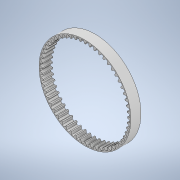
# Autodesk Inventor part: Zahnriemen
Saved by Autodesk Inventor 2021 (Build 250183000, 183)
## iProperties
Created: 2021-08-21
Part Number: Zahnriemen
Material: Generisch
Document SubType Name: Modeling
Designer: stroh
Density: 1 g/cm^3
Appearance: Vorgabe
Author: stroh
Autodesk Inventor part; units mm, degrees
ref_plane "YZ Plane" through (0, 0, 0) normal (1, 0, 0) x (0, 1, 0)
ref_plane "XZ Plane" through (0, 0, 0) normal (0, 1, 0) x (-1, 0, 0)
ref_plane "XY Plane" through (0, 0, 0) normal (0, 0, 1) x (1, 0, 0)
sketch "Skizze2" plane through (0, 0, 0) normal (0, 0, 1) x (1, 0, 0)
  circle A0 centre (0, 0) radius 44.5634
  line L0 (1.5, 44.5381) -> (0.5, 42.0381)
  line L1 (0.5, 42.0381) -> (-0.5, 42.0381)
  line L2 (-0.5, 42.0381) -> (-1.5, 44.5381)
  arc A1 (1.5, 44.5381) -> (-1.5, 44.5381) centre (0, 0) ccw
  circle A2 centre (0, 0) radius 45.5
  arc A3 (-3.4961, 44.426) -> (-6.4773, 44.0901) centre (0, 0) ccw
  line L3 (-5.2036, 41.7178) -> (-6.4773, 44.0901)
  line L4 (-4.2099, 41.8298) -> (-5.2036, 41.7178)
  line L5 (-3.4961, 44.426) -> (-4.2099, 41.8298)
  arc A4 (-8.4483, 43.7553) -> (-11.3731, 43.0877) centre (0, 0) ccw
  line L6 (-9.8418, 40.8729) -> (-11.3731, 43.0877)
  line L7 (-8.8669, 41.0954) -> (-9.8418, 40.8729)
  line L8 (-8.4483, 43.7553) -> (-8.8669, 41.0954)
  arc A5 (-13.2942, 42.5342) -> (-16.1258, 41.5434) centre (0, 0) ccw
  line L9 (-14.3563, 39.514) -> (-16.1258, 41.5434)
  line L10 (-13.4124, 39.8442) -> (-14.3563, 39.514)
  line L11 (-13.2942, 42.5342) -> (-13.4124, 39.8442)
  arc A6 (-17.9729, 40.7783) -> (-20.6758, 39.4766) centre (0, 0) ccw
  line L12 (-18.6901, 37.6581) -> (-20.6758, 39.4766)
  line L13 (-17.7892, 38.092) -> (-18.6901, 37.6581)
  line L14 (-17.9729, 40.7783) -> (-17.7892, 38.092)
  arc A7 (-22.4256, 38.5096) -> (-24.9658, 36.9135) centre (0, 0) ccw
  line L15 (-22.789, 35.3287) -> (-24.9658, 36.9135)
  line L16 (-21.9423, 35.8607) -> (-22.789, 35.3287)
  line L17 (-22.4256, 38.5096) -> (-21.9423, 35.8607)
  arc A8 (-26.5963, 35.7565) -> (-28.9418, 33.8861) centre (0, 0) ccw
  line L18 (-26.6013, 32.555) -> (-28.9418, 33.8861)
  line L19 (-25.8194, 33.1785) -> (-26.6013, 32.555)
  line L20 (-26.5963, 35.7565) -> (-25.8194, 33.1785)
  arc A9 (-30.4326, 32.5539) -> (-32.5539, 30.4326) centre (0, 0) ccw
  line L21 (-30.079, 29.3719) -> (-32.5539, 30.4326)
  line L22 (-29.3719, 30.079) -> (-30.079, 29.3719)
  line L23 (-30.4326, 32.5539) -> (-29.3719, 30.079)
  arc A10 (-33.8861, 28.9418) -> (-35.7565, 26.5963) centre (0, 0) ccw
  line L24 (-33.1785, 25.8194) -> (-35.7565, 26.5963)
  line L25 (-32.555, 26.6013) -> (-33.1785, 25.8194)
  line L26 (-33.8861, 28.9418) -> (-32.555, 26.6013)
  arc A11 (-36.9135, 24.9658) -> (-38.5096, 22.4256) centre (0, 0) ccw
  line L27 (-35.8607, 21.9423) -> (-38.5096, 22.4256)
  line L28 (-35.3287, 22.789) -> (-35.8607, 21.9423)
  line L29 (-36.9135, 24.9658) -> (-35.3287, 22.789)
  arc A12 (-39.4766, 20.6758) -> (-40.7783, 17.9729) centre (0, 0) ccw
  line L30 (-38.092, 17.7892) -> (-40.7783, 17.9729)
  line L31 (-37.6581, 18.6901) -> (-38.092, 17.7892)
  line L32 (-39.4766, 20.6758) -> (-37.6581, 18.6901)
  arc A13 (-41.5434, 16.1258) -> (-42.5342, 13.2942) centre (0, 0) ccw
  line L33 (-39.8442, 13.4124) -> (-42.5342, 13.2942)
  line L34 (-39.514, 14.3563) -> (-39.8442, 13.4124)
  line L35 (-41.5434, 16.1258) -> (-39.514, 14.3563)
  arc A14 (-43.0877, 11.3731) -> (-43.7553, 8.4483) centre (0, 0) ccw
  line L36 (-41.0954, 8.8669) -> (-43.7553, 8.4483)
  line L37 (-40.8729, 9.8418) -> (-41.0954, 8.8669)
  line L38 (-43.0877, 11.3731) -> (-40.8729, 9.8418)
  arc A15 (-44.0901, 6.4773) -> (-44.426, 3.4961) centre (0, 0) ccw
  line L39 (-41.8298, 4.2099) -> (-44.426, 3.4961)
  line L40 (-41.7178, 5.2036) -> (-41.8298, 4.2099)
  line L41 (-44.0901, 6.4773) -> (-41.7178, 5.2036)
  arc A16 (-44.5381, 1.5) -> (-44.5381, -1.5) centre (0, 0) ccw
  line L42 (-42.0381, -0.5) -> (-44.5381, -1.5)
  line L43 (-42.0381, 0.5) -> (-42.0381, -0.5)
  line L44 (-44.5381, 1.5) -> (-42.0381, 0.5)
  arc A17 (-44.426, -3.4961) -> (-44.0901, -6.4773) centre (0, 0) ccw
  line L45 (-41.7178, -5.2036) -> (-44.0901, -6.4773)
  line L46 (-41.8298, -4.2099) -> (-41.7178, -5.2036)
  line L47 (-44.426, -3.4961) -> (-41.8298, -4.2099)
  arc A18 (-43.7553, -8.4483) -> (-43.0877, -11.3731) centre (0, 0) ccw
  line L48 (-40.8729, -9.8418) -> (-43.0877, -11.3731)
  line L49 (-41.0954, -8.8669) -> (-40.8729, -9.8418)
  line L50 (-43.7553, -8.4483) -> (-41.0954, -8.8669)
  arc A19 (-42.5342, -13.2942) -> (-41.5434, -16.1258) centre (0, 0) ccw
  line L51 (-39.514, -14.3563) -> (-41.5434, -16.1258)
  line L52 (-39.8442, -13.4124) -> (-39.514, -14.3563)
  line L53 (-42.5342, -13.2942) -> (-39.8442, -13.4124)
  arc A20 (-40.7783, -17.9729) -> (-39.4766, -20.6758) centre (0, 0) ccw
  line L54 (-37.6581, -18.6901) -> (-39.4766, -20.6758)
  line L55 (-38.092, -17.7892) -> (-37.6581, -18.6901)
  line L56 (-40.7783, -17.9729) -> (-38.092, -17.7892)
  arc A21 (-38.5096, -22.4256) -> (-36.9135, -24.9658) centre (0, 0) ccw
  line L57 (-35.3287, -22.789) -> (-36.9135, -24.9658)
  line L58 (-35.8607, -21.9423) -> (-35.3287, -22.789)
  line L59 (-38.5096, -22.4256) -> (-35.8607, -21.9423)
  arc A22 (-35.7565, -26.5963) -> (-33.8861, -28.9418) centre (0, 0) ccw
  line L60 (-32.555, -26.6013) -> (-33.8861, -28.9418)
  line L61 (-33.1785, -25.8194) -> (-32.555, -26.6013)
  line L62 (-35.7565, -26.5963) -> (-33.1785, -25.8194)
  arc A23 (-32.5539, -30.4326) -> (-30.4326, -32.5539) centre (0, 0) ccw
  line L63 (-29.3719, -30.079) -> (-30.4326, -32.5539)
  line L64 (-30.079, -29.3719) -> (-29.3719, -30.079)
  line L65 (-32.5539, -30.4326) -> (-30.079, -29.3719)
  arc A24 (-28.9418, -33.8861) -> (-26.5963, -35.7565) centre (0, 0) ccw
  line L66 (-25.8194, -33.1785) -> (-26.5963, -35.7565)
  line L67 (-26.6013, -32.555) -> (-25.8194, -33.1785)
  line L68 (-28.9418, -33.8861) -> (-26.6013, -32.555)
  arc A25 (-24.9658, -36.9135) -> (-22.4256, -38.5096) centre (0, 0) ccw
  line L69 (-21.9423, -35.8607) -> (-22.4256, -38.5096)
  line L70 (-22.789, -35.3287) -> (-21.9423, -35.8607)
  line L71 (-24.9658, -36.9135) -> (-22.789, -35.3287)
  arc A26 (-20.6758, -39.4766) -> (-17.9729, -40.7783) centre (0, 0) ccw
  line L72 (-17.7892, -38.092) -> (-17.9729, -40.7783)
  line L73 (-18.6901, -37.6581) -> (-17.7892, -38.092)
  line L74 (-20.6758, -39.4766) -> (-18.6901, -37.6581)
  arc A27 (-16.1258, -41.5434) -> (-13.2942, -42.5342) centre (0, 0) ccw
  line L75 (-13.4124, -39.8442) -> (-13.2942, -42.5342)
  line L76 (-14.3563, -39.514) -> (-13.4124, -39.8442)
  line L77 (-16.1258, -41.5434) -> (-14.3563, -39.514)
  arc A28 (-11.3731, -43.0877) -> (-8.4483, -43.7553) centre (0, 0) ccw
  line L78 (-8.8669, -41.0954) -> (-8.4483, -43.7553)
  line L79 (-9.8418, -40.8729) -> (-8.8669, -41.0954)
  line L80 (-11.3731, -43.0877) -> (-9.8418, -40.8729)
  arc A29 (-6.4773, -44.0901) -> (-3.4961, -44.426) centre (0, 0) ccw
  line L81 (-4.2099, -41.8298) -> (-3.4961, -44.426)
  line L82 (-5.2036, -41.7178) -> (-4.2099, -41.8298)
  line L83 (-6.4773, -44.0901) -> (-5.2036, -41.7178)
  arc A30 (-1.5, -44.5381) -> (1.5, -44.5381) centre (0, 0) ccw
  line L84 (0.5, -42.0381) -> (1.5, -44.5381)
  line L85 (-0.5, -42.0381) -> (0.5, -42.0381)
  line L86 (-1.5, -44.5381) -> (-0.5, -42.0381)
  arc A31 (3.4961, -44.426) -> (6.4773, -44.0901) centre (0, 0) ccw
  line L87 (5.2036, -41.7178) -> (6.4773, -44.0901)
  line L88 (4.2099, -41.8298) -> (5.2036, -41.7178)
  line L89 (3.4961, -44.426) -> (4.2099, -41.8298)
  arc A32 (8.4483, -43.7553) -> (11.3731, -43.0877) centre (0, 0) ccw
  line L90 (9.8418, -40.8729) -> (11.3731, -43.0877)
  line L91 (8.8669, -41.0954) -> (9.8418, -40.8729)
  line L92 (8.4483, -43.7553) -> (8.8669, -41.0954)
  arc A33 (13.2942, -42.5342) -> (16.1258, -41.5434) centre (0, 0) ccw
  line L93 (14.3563, -39.514) -> (16.1258, -41.5434)
  line L94 (13.4124, -39.8442) -> (14.3563, -39.514)
  line L95 (13.2942, -42.5342) -> (13.4124, -39.8442)
  arc A34 (17.9729, -40.7783) -> (20.6758, -39.4766) centre (0, 0) ccw
  line L96 (18.6901, -37.6581) -> (20.6758, -39.4766)
  line L97 (17.7892, -38.092) -> (18.6901, -37.6581)
  line L98 (17.9729, -40.7783) -> (17.7892, -38.092)
  arc A35 (22.4256, -38.5096) -> (24.9658, -36.9135) centre (0, 0) ccw
  line L99 (22.789, -35.3287) -> (24.9658, -36.9135)
  line L100 (21.9423, -35.8607) -> (22.789, -35.3287)
  line L101 (22.4256, -38.5096) -> (21.9423, -35.8607)
  arc A36 (26.5963, -35.7565) -> (28.9418, -33.8861) centre (0, 0) ccw
  line L102 (26.6013, -32.555) -> (28.9418, -33.8861)
  line L103 (25.8194, -33.1785) -> (26.6013, -32.555)
  line L104 (26.5963, -35.7565) -> (25.8194, -33.1785)
  arc A37 (30.4326, -32.5539) -> (32.5539, -30.4326) centre (0, 0) ccw
  line L105 (30.079, -29.3719) -> (32.5539, -30.4326)
  line L106 (29.3719, -30.079) -> (30.079, -29.3719)
  line L107 (30.4326, -32.5539) -> (29.3719, -30.079)
  arc A38 (33.8861, -28.9418) -> (35.7565, -26.5963) centre (0, 0) ccw
  line L108 (33.1785, -25.8194) -> (35.7565, -26.5963)
  line L109 (32.555, -26.6013) -> (33.1785, -25.8194)
  line L110 (33.8861, -28.9418) -> (32.555, -26.6013)
  arc A39 (36.9135, -24.9658) -> (38.5096, -22.4256) centre (0, 0) ccw
  line L111 (35.8607, -21.9423) -> (38.5096, -22.4256)
  line L112 (35.3287, -22.789) -> (35.8607, -21.9423)
  line L113 (36.9135, -24.9658) -> (35.3287, -22.789)
  arc A40 (39.4766, -20.6758) -> (40.7783, -17.9729) centre (0, 0) ccw
  line L114 (38.092, -17.7892) -> (40.7783, -17.9729)
  line L115 (37.6581, -18.6901) -> (38.092, -17.7892)
  line L116 (39.4766, -20.6758) -> (37.6581, -18.6901)
  arc A41 (41.5434, -16.1258) -> (42.5342, -13.2942) centre (0, 0) ccw
  line L117 (39.8442, -13.4124) -> (42.5342, -13.2942)
  line L118 (39.514, -14.3563) -> (39.8442, -13.4124)
  line L119 (41.5434, -16.1258) -> (39.514, -14.3563)
  arc A42 (43.0877, -11.3731) -> (43.7553, -8.4483) centre (0, 0) ccw
  line L120 (41.0954, -8.8669) -> (43.7553, -8.4483)
  line L121 (40.8729, -9.8418) -> (41.0954, -8.8669)
  line L122 (43.0877, -11.3731) -> (40.8729, -9.8418)
  arc A43 (44.0901, -6.4773) -> (44.426, -3.4961) centre (0, 0) ccw
  line L123 (41.8298, -4.2099) -> (44.426, -3.4961)
  line L124 (41.7178, -5.2036) -> (41.8298, -4.2099)
  line L125 (44.0901, -6.4773) -> (41.7178, -5.2036)
  arc A44 (44.5381, -1.5) -> (44.5381, 1.5) centre (0, 0) ccw
  line L126 (42.0381, 0.5) -> (44.5381, 1.5)
  line L127 (42.0381, -0.5) -> (42.0381, 0.5)
  line L128 (44.5381, -1.5) -> (42.0381, -0.5)
  arc A45 (44.426, 3.4961) -> (44.0901, 6.4773) centre (0, 0) ccw
  line L129 (41.7178, 5.2036) -> (44.0901, 6.4773)
  line L130 (41.8298, 4.2099) -> (41.7178, 5.2036)
  line L131 (44.426, 3.4961) -> (41.8298, 4.2099)
  arc A46 (43.7553, 8.4483) -> (43.0877, 11.3731) centre (0, 0) ccw
  line L132 (40.8729, 9.8418) -> (43.0877, 11.3731)
  line L133 (41.0954, 8.8669) -> (40.8729, 9.8418)
  line L134 (43.7553, 8.4483) -> (41.0954, 8.8669)
  arc A47 (42.5342, 13.2942) -> (41.5434, 16.1258) centre (0, 0) ccw
  line L135 (39.514, 14.3563) -> (41.5434, 16.1258)
  line L136 (39.8442, 13.4124) -> (39.514, 14.3563)
  line L137 (42.5342, 13.2942) -> (39.8442, 13.4124)
  arc A48 (40.7783, 17.9729) -> (39.4766, 20.6758) centre (0, 0) ccw
  line L138 (37.6581, 18.6901) -> (39.4766, 20.6758)
  line L139 (38.092, 17.7892) -> (37.6581, 18.6901)
  line L140 (40.7783, 17.9729) -> (38.092, 17.7892)
  arc A49 (38.5096, 22.4256) -> (36.9135, 24.9658) centre (0, 0) ccw
  line L141 (35.3287, 22.789) -> (36.9135, 24.9658)
  line L142 (35.8607, 21.9423) -> (35.3287, 22.789)
  line L143 (38.5096, 22.4256) -> (35.8607, 21.9423)
  arc A50 (35.7565, 26.5963) -> (33.8861, 28.9418) centre (0, 0) ccw
  line L144 (32.555, 26.6013) -> (33.8861, 28.9418)
  line L145 (33.1785, 25.8194) -> (32.555, 26.6013)
  line L146 (35.7565, 26.5963) -> (33.1785, 25.8194)
  arc A51 (32.5539, 30.4326) -> (30.4326, 32.5539) centre (0, 0) ccw
  line L147 (29.3719, 30.079) -> (30.4326, 32.5539)
  line L148 (30.079, 29.3719) -> (29.3719, 30.079)
  line L149 (32.5539, 30.4326) -> (30.079, 29.3719)
  arc A52 (28.9418, 33.8861) -> (26.5963, 35.7565) centre (0, 0) ccw
  line L150 (25.8194, 33.1785) -> (26.5963, 35.7565)
  line L151 (26.6013, 32.555) -> (25.8194, 33.1785)
  line L152 (28.9418, 33.8861) -> (26.6013, 32.555)
  arc A53 (24.9658, 36.9135) -> (22.4256, 38.5096) centre (0, 0) ccw
  line L153 (21.9423, 35.8607) -> (22.4256, 38.5096)
  line L154 (22.789, 35.3287) -> (21.9423, 35.8607)
  line L155 (24.9658, 36.9135) -> (22.789, 35.3287)
  arc A54 (20.6758, 39.4766) -> (17.9729, 40.7783) centre (0, 0) ccw
  line L156 (17.7892, 38.092) -> (17.9729, 40.7783)
  line L157 (18.6901, 37.6581) -> (17.7892, 38.092)
  line L158 (20.6758, 39.4766) -> (18.6901, 37.6581)
  arc A55 (16.1258, 41.5434) -> (13.2942, 42.5342) centre (0, 0) ccw
  line L159 (13.4124, 39.8442) -> (13.2942, 42.5342)
  line L160 (14.3563, 39.514) -> (13.4124, 39.8442)
  line L161 (16.1258, 41.5434) -> (14.3563, 39.514)
  arc A56 (11.3731, 43.0877) -> (8.4483, 43.7553) centre (0, 0) ccw
  line L162 (8.8669, 41.0954) -> (8.4483, 43.7553)
  line L163 (9.8418, 40.8729) -> (8.8669, 41.0954)
  line L164 (11.3731, 43.0877) -> (9.8418, 40.8729)
  arc A57 (6.4773, 44.0901) -> (3.4961, 44.426) centre (0, 0) ccw
  line L165 (4.2099, 41.8298) -> (3.4961, 44.426)
  line L166 (5.2036, 41.7178) -> (4.2099, 41.8298)
  line L167 (6.4773, 44.0901) -> (5.2036, 41.7178)
  point P0 (44.5381, 1.5)
  point P1 (44.5381, -1.5)
  point P2 (44.426, -3.4961)
  point P3 (44.0901, -6.4773)
  point P4 (43.7553, -8.4483)
  point P5 (43.0877, -11.3731)
  point P6 (42.5342, -13.2942)
  point P7 (41.5434, -16.1258)
  point P8 (40.7783, -17.9729)
  point P9 (39.4766, -20.6758)
  point P10 (38.5096, -22.4256)
  point P11 (36.9135, -24.9658)
  point P12 (35.7565, -26.5963)
  point P13 (33.8861, -28.9418)
  point P14 (32.5539, -30.4326)
  point P15 (30.4326, -32.5539)
  point P16 (28.9418, -33.8861)
  point P17 (26.5963, -35.7565)
  point P18 (24.9658, -36.9135)
  point P19 (22.4256, -38.5096)
  point P20 (20.6758, -39.4766)
  point P21 (17.9729, -40.7783)
  point P22 (16.1258, -41.5434)
  point P23 (13.2942, -42.5342)
  point P24 (11.3731, -43.0877)
  point P25 (8.4483, -43.7553)
  point P26 (6.4773, -44.0901)
  point P27 (3.4961, -44.426)
  point P28 (1.5, -44.5381)
  point P29 (-1.5, -44.5381)
  point P30 (-3.4961, -44.426)
  point P31 (-6.4773, -44.0901)
  point P32 (-8.4483, -43.7553)
  point P33 (-11.3731, -43.0877)
  point P34 (-13.2942, -42.5342)
  point P35 (-16.1258, -41.5434)
  point P36 (-17.9729, -40.7783)
  point P37 (-20.6758, -39.4766)
  point P38 (-22.4256, -38.5096)
  point P39 (-24.9658, -36.9135)
  point P40 (-26.5963, -35.7565)
  point P41 (-28.9418, -33.8861)
  point P42 (-30.4326, -32.5539)
  point P43 (-32.5539, -30.4326)
  point P44 (-33.8861, -28.9418)
  point P45 (-35.7565, -26.5963)
  point P46 (-36.9135, -24.9658)
  point P47 (-38.5096, -22.4256)
  point P48 (-39.4766, -20.6758)
  point P49 (-40.7783, -17.9729)
  point P50 (-41.5434, -16.1258)
  point P51 (-42.5342, -13.2942)
  point P52 (-43.0877, -11.3731)
  point P53 (-43.7553, -8.4483)
  point P54 (-44.0901, -6.4773)
  point P55 (-44.426, -3.4961)
  point P56 (-44.5381, -1.5)
  point P57 (-44.5381, 1.5)
  point P58 (-44.426, 3.4961)
  point P59 (-44.0901, 6.4773)
  point P60 (-43.7553, 8.4483)
  point P61 (-43.0877, 11.3731)
  point P62 (-42.5342, 13.2942)
  point P63 (-41.5434, 16.1258)
  point P64 (-40.7783, 17.9729)
  point P65 (-39.4766, 20.6758)
  point P66 (-38.5096, 22.4256)
  point P67 (-36.9135, 24.9658)
  point P68 (-35.7565, 26.5963)
  point P69 (-33.8861, 28.9418)
  point P70 (-32.5539, 30.4326)
  point P71 (-30.4326, 32.5539)
  point P72 (-28.9418, 33.8861)
  point P73 (-26.5963, 35.7565)
  point P74 (-24.9658, 36.9135)
  point P75 (-22.4256, 38.5096)
  point P76 (-20.6758, 39.4766)
  point P77 (-17.9729, 40.7783)
  point P78 (-16.1258, 41.5434)
  point P79 (-13.2942, 42.5342)
  point P80 (-11.3731, 43.0877)
  point P81 (-8.4483, 43.7553)
  point P82 (-6.4773, 44.0901)
  point P83 (-3.4961, 44.426)
  point P84 (3.4961, 44.426)
  point P85 (6.4773, 44.0901)
  point P86 (8.4483, 43.7553)
  point P87 (11.3731, 43.0877)
  point P88 (13.2942, 42.5342)
  point P89 (16.1258, 41.5434)
  point P90 (17.9729, 40.7783)
  point P91 (20.6758, 39.4766)
  point P92 (22.4256, 38.5096)
  point P93 (24.9658, 36.9135)
  point P94 (26.5963, 35.7565)
  point P95 (28.9418, 33.8861)
  point P96 (30.4326, 32.5539)
  point P97 (32.5539, 30.4326)
  point P98 (33.8861, 28.9418)
  point P99 (35.7565, 26.5963)
  point P100 (36.9135, 24.9658)
  point P101 (38.5096, 22.4256)
  point P102 (39.4766, 20.6758)
  point P103 (40.7783, 17.9729)
  point P104 (41.5434, 16.1258)
  point P105 (42.5342, 13.2942)
  point P106 (43.0877, 11.3731)
  point P107 (43.7553, 8.4483)
  point P108 (44.0901, 6.4773)
  point P109 (44.426, 3.4961)
  dimension "d16" = 89.1268
  dimension "d17" = 3
  dimension "d18" = 1
  dimension "d20" = 0.5
  dimension "d25" = 91
  dimension "d31" = 360
  constraints: 336 end point, 112 point on circle, 57 centre point, 1 coincident, 509 other
  measures "d17" distance of L2.end L0.start
  measures "d18" distance of L0.end L1.end
  measures "d20" horizontal distance of point (0, 0) L0.end
  measures "d25" diameter of A2
extrude "Extrusion3" add sketch "Skizze2" along normal blind 10 contours A0 L128 L127 L126 | L131 L130 L129 A0 | A0 L125 L124 L123 | L134 L133 L132 A0 | A0 L122 L121 L120 | L137 L136 L135 A0 | A0 L119 L118 L117 | L140 L139 L138 A0 | A0 L116 L115 L114 | L143 L142 L141 A0 | A0 L113 L112 L111 | L146 L145 L144 A0 | A0 L110 L109 L108 | L149 L148 L147 A0 | A0 L107 L106 L105 | L152 L151 L150 A0 | A0 L104 L103 L102 | L155 L154 L153 A0 | A0 L101 L100 L99 | L158 L157 L156 A0 | A0 L98 L97 L96 | L161 L160 L159 A0 | A0 L95 L94 L93 | L164 L163 L162 A0 | A0 L92 L91 L90 | L167 L166 L165 A0 | A0 L89 L88 L87 | L0 L1 L2 A0 | A0 L86 L85 L84 | L5 L4 L3 A0 | A0 L83 L82 L81 | L8 L7 L6 A0 | A0 L80 L79 L78 | L11 L10 L9 A0 | A0 L77 L76 L75 | L14 L13 L12 A0 | A0 L74 L73 L72 | L17 L16 L15 A0 | A0 L71 L70 L69 | L20 L19 L18 A0 | A0 L68 L67 L66 | L23 L22 L21 A0 | A0 L65 L64 L63 | L26 L25 L24 A0 | A0 L62 L61 L60 | L29 L28 L27 A0 | A0 L59 L58 L57 | L32 L31 L30 A0 | A0 L56 L55 L54 | L35 L34 L33 A0 | A0 L53 L52 L51 | L38 L37 L36 A0 | A0 L50 L49 L48 | L41 L40 L39 A0 | A0 L47 L46 L45 | L44 L43 L42 A0 | A2
